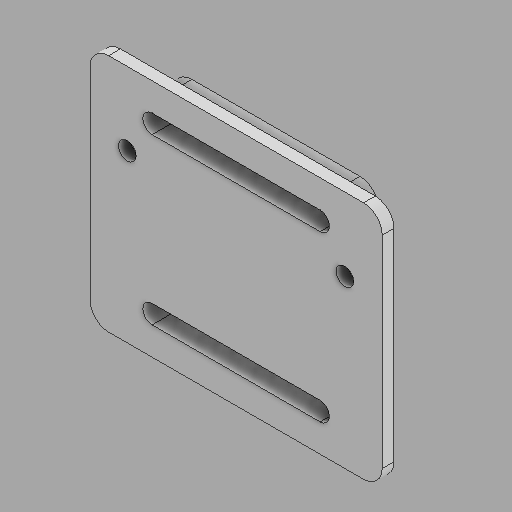
# Autodesk Inventor part: RC_CAR_ARDUINO_PLATE
Saved by Autodesk Inventor 2025.2 (Build 292293000, 293)
## iProperties
Created: 2026-01-02
Part Number: RC_CAR_ARDUINO_PLATE
Material: Generic
Document SubType Name: Modeling
Designer: Ben
Density: 1 g/cm^3
Appearance: Default
Author: Ben
Autodesk Inventor part; units mm, degrees
ref_plane "YZ Plane" through (0, 0, 0) normal (1, 0, 0) x (0, 1, 0)
ref_plane "XZ Plane" through (0, 0, 0) normal (0, 1, 0) x (-1, 0, 0)
ref_plane "XY Plane" through (0, 0, 0) normal (0, 0, 1) x (1, 0, 0)
sketch "Sketch1" plane through (0, 0, 0) normal (0, 0, 1) x (1, 0, 0)
  line L0 (-24.85, -20.36) -> (24.85, -20.36)
  line L1 (24.85, -20.36) -> (24.85, 20.36)
  line L2 (24.85, 20.36) -> (-24.85, 20.36)
  line L3 (-24.85, 20.36) -> (-24.85, -20.36)
  line L4 (-24.85, -20.36) -> (24.85, 20.36) construction
  line L5 (24.85, -20.36) -> (-24.85, 20.36) construction
  point P0 (0, 0)
  dimension "d0" = 49.7
  dimension "d1" = 40.72
  constraints: 12 end point, 2 midpoint, 2 parallel, 1 horizontal, 1 perpendicular
  measures "d0" distance of L1.end L2.end
  measures "d1" distance of L2.end L0.start
extrude "Extrusion1" add sketch "Sketch1" along normal blind 2
sketch "Sketch3" plane through (0, 0, 0) normal (0, 0, -1) x (-1, 0, 0)
  line L0 (24.85, 20.36) -> (24.85, -20.36) projected
  line L1 (14.2875, -14.01) -> (-14.2875, -14.01) construction
  line L2 (14.2875, -10.835) -> (-14.2875, -10.835)
  line L3 (-14.2875, -17.185) -> (14.2875, -17.185)
  arc A0 (14.2875, -17.185) -> (14.2875, -10.835) centre (14.2875, -14.01) ccw
  arc A1 (-14.2875, -10.835) -> (-14.2875, -17.185) centre (-14.2875, -14.01) ccw
  line L4 (0, -28.504) -> (0, 28.504) projected
  line L5 (34.79, 0) -> (-34.79, 0) projected
  line L6 (14.2875, 14.01) -> (-14.2875, 14.01) construction
  line L7 (14.2875, 17.185) -> (-14.2875, 17.185)
  line L8 (-14.2875, 10.835) -> (14.2875, 10.835)
  arc A2 (14.2875, 10.835) -> (14.2875, 17.185) centre (14.2875, 14.01) ccw
  arc A3 (-14.2875, 17.185) -> (-14.2875, 10.835) centre (-14.2875, 14.01) ccw
  point P0 (0, 0)
  point P1 (0, -14.01)
  point P2 (0, 14.01)
  dimension "d28" = 3.175
  dimension "d29" = 28.02
  dimension "d30" = 28.575
  constraints: 16 end point, 8 point on circle, 8 tangent, 4 centre point, 3 parallel, 2 midpoint, 1 horizontal, 1 symmetric about line, 2 other
  measures "d28" radius of A1
  measures "d29" distance between parallel lines of L6 L1
  measures "d30" distance of L3.start L3.end
sketch "Sketch5" plane through (0, 0, 0) normal (0, 0, -1) x (-1, 0, 0)
  line L0 (0, -28.504) -> (0, 28.504) projected
  line L1 (34.79, 0) -> (-34.79, 0) projected
  point P0 (0, 0)
  point P1 (-18.5, 7.9375)
  point P2 (18.5, 7.9375)
  dimension "d17" = 37
  dimension "d26" = 7.9375
  constraints: 1 horizontal alignment, 1 symmetric about line
  measures "d17" distance of point (18.5, 7.938) point (-18.5, 7.938)
  measures "d26" distance from line of L1 point (-18.5, 7.938)
hole "Hole1" at (18.5, 7.9375, 0) at (-18.5, 7.9375, 0) direction (0, 0, 1) diameter 3 depth 2
fillet "Fillet1" radius 3.175 4 edges at (24.85, -20.36, 1) (24.85, 20.36, 1) (-24.85, 20.36, 1) (-24.85, -20.36, 1)
extrude "Extrusion4" add sketch "Sketch3" along normal blind 4.7625
sketch "Sketch6" plane through (0, 0, -4.7625) normal (0, 0, -1) x (-1, 0, 0)
  line L0 (14.2875, -10.835) -> (-14.2875, -10.835) projected
  arc A0 (-14.2875, -10.835) -> (-14.2875, -17.185) centre (-14.2875, -14.01) ccw projected
  line L1 (-14.2875, -17.185) -> (14.2875, -17.185) projected
  arc A1 (14.2875, -17.185) -> (14.2875, -10.835) centre (14.2875, -14.01) ccw projected
  line L2 (14.2875, 17.185) -> (-14.2875, 17.185) projected
  arc A2 (-14.2875, 17.185) -> (-14.2875, 10.835) centre (-14.2875, 14.01) ccw projected
  line L3 (-14.2875, 10.835) -> (14.2875, 10.835) projected
  arc A3 (14.2875, 10.835) -> (14.2875, 17.185) centre (14.2875, 14.01) ccw projected
  line L4 (14.2875, -14.01) -> (-14.2875, -14.01) construction
  line L5 (14.2875, -12.4225) -> (-14.2875, -12.4225)
  line L6 (-14.2875, -15.5975) -> (14.2875, -15.5975)
  arc A4 (14.2875, -15.5975) -> (14.2875, -12.4225) centre (14.2875, -14.01) ccw
  arc A5 (-14.2875, -12.4225) -> (-14.2875, -15.5975) centre (-14.2875, -14.01) ccw
  line L7 (14.2875, 14.01) -> (-14.2875, 14.01) construction
  line L8 (14.2875, 15.5975) -> (-14.2875, 15.5975)
  line L9 (-14.2875, 12.4225) -> (14.2875, 12.4225)
  arc A6 (14.2875, 12.4225) -> (14.2875, 15.5975) centre (14.2875, 14.01) ccw
  arc A7 (-14.2875, 15.5975) -> (-14.2875, 12.4225) centre (-14.2875, 14.01) ccw
  point P0 (0, 0)
  point P1 (0, -14.01)
  point P2 (0, 14.01)
  dimension "d33" = 1.5875
  constraints: 16 end point, 8 point on circle, 8 tangent, 4 centre point, 3 parallel, 2 midpoint, 1 equal radius, 1 horizontal
  measures "d33" radial gap between concentric circles of A1 A4
extrude "Extrusion5" cut sketch "Sketch6" along normal through all both and the other way through all contours A4 L6 A5 L5 | A6 L9 A7 L8
body "Solid1"
